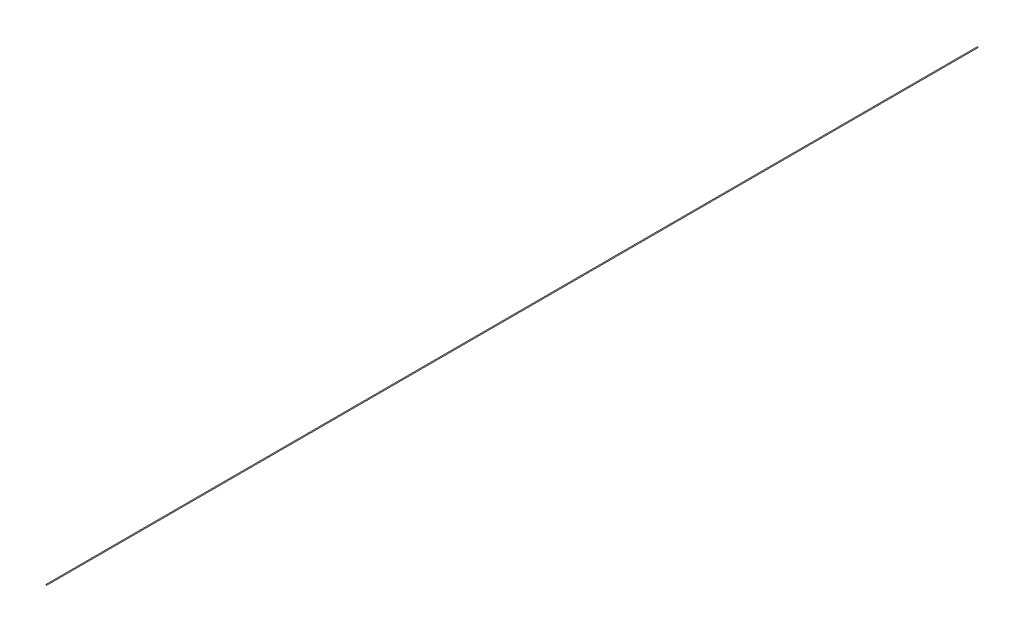
# Autodesk Inventor part: kev-central
Saved by Autodesk Inventor 2013 SP2 (Build 170200200, 200)
## iProperties
Company: HERA Project
Created: 2013-05-28
Part Number: kev-central
Material: Polyethylene, High Density
Document SubType Name: Modeling
Designer: David DeBoer
Density: 1 g/cm^3
Description: Kevlar central support
Author: David DeBoer
Title: Kevlar central support
Autodesk Inventor part; units mm, degrees
ref_plane "YZ Plane" through (0, 0, 0) normal (1, 0, 0) x (0, 1, 0)
ref_plane "XZ Plane" through (0, 0, 0) normal (0, 1, 0) x (-1, 0, 0)
ref_plane "XY Plane" through (0, 0, 0) normal (0, 0, 1) x (1, 0, 0)
sketch "Sketch1" plane through (0, 0, 0) normal (0, 0, 1) x (1, 0, 0)
  circle A0 centre (0, 0) radius 3.81
  dimension "d0" = 7.62
  constraints: 1 centre point, 1 coincident
  measures "d0" diameter of A0
extrude "Extrusion1" add sketch "Sketch1" along normal blind 8128
body "Solid1"
